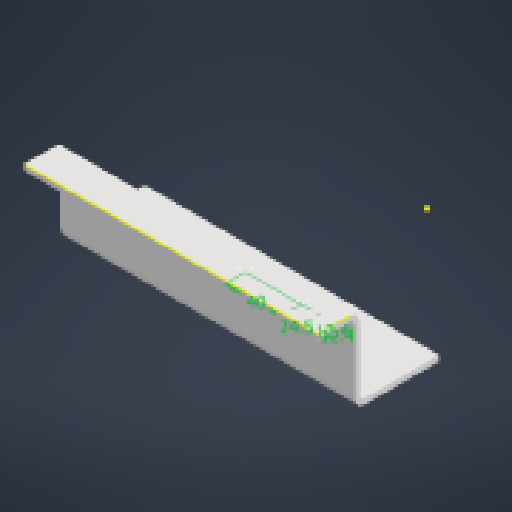
# Autodesk Inventor part: Bottom joint housing R
Saved by Autodesk Inventor 2026.3 (Build 303398000, 398)
## iProperties
Created: 2026-08-05
Part Number: Bottom joint housing R
Material: Generic
Document SubType Name: Sheet Metal
Designer: matot
Density: 1 g/cm^3
Sheet Metal Rule: Default_mm
Appearance: Default
Author: matot
Autodesk Inventor part; units mm, degrees
ref_plane "YZ Plane" through (0, 0, 0) normal (1, 0, 0) x (0, 1, 0)
ref_plane "XZ Plane" through (0, 0, 0) normal (0, 1, 0) x (-1, 0, 0)
ref_plane "XY Plane" through (0, 0, 0) normal (0, 0, 1) x (1, 0, 0)
sketch "Sketch1" plane through (0, 0, 0) normal (0, 1, 0) x (-1, 0, 0)
  line L0 (171.8333, 340.8333) -> (-39.1667, 340.8333)
  line L1 (-39.1667, 340.8333) -> (-39.1667, -59.1667)
  line L2 (-39.1667, -59.1667) -> (171.8333, -59.1667)
  line L3 (171.8333, -59.1667) -> (171.8333, 340.8333)
  point P0 (0, 0)
  dimension "d0" = 400
  dimension "d1" = 211
  measures "d0" distance of L0.end L1.end
  measures "d1" distance of L1.end L2.end
extrude "Plate1" add sketch "Sketch1" along normal blind 4
sketch "Sketch2" plane through (0, 4, 0) normal (0, 1, 0) x (1, 0, 0)
  line L0 (-171.8333, 59.1667) -> (-171.8333, -340.8333) projected
  line L1 (-171.8333, -137.1069) -> (39.1667, -137.1069)
  line L2 (-171.8333, -37.1069) -> (39.1667, -37.1069)
  line L3 (39.1667, -37.1069) -> (39.1667, -37.1069)
  line L4 (39.1667, 59.1667) -> (39.1667, -340.8333) projected
  point P0 (0, 0)
  dimension "d3" = 100
  dimension "d4" = 211
  dimension "d5" = 211
  constraints: 6 end point, 3 perpendicular, 2 point on line, 1 horizontal
  measures "d3" distance between parallel lines of L2 L1
  measures "d4" distance of L2.start L2.end
  measures "d5" distance of L1.start L1.end
fold "Fold1" angle 90 bend radius 4 thickness 4 k factor 0.44 line from (-171.8333, 4, 37.1069) to (39.1667, 4, 37.1069) line at bend centre moving side (0, 0, -1) folds toward (0, 1, 0)
sketch "Sketch3" plane through (0, 0, 0) normal (0, -1, 0) x (1, 0, 0)
  line L0 (39.1667, 41.6308) -> (39.1667, 340.8333) projected
  line L1 (39.1667, 90.6308) -> (-171.8333, 90.6308)
  line L2 (39.1667, 33.6308) -> (-171.8333, 33.6308) projected
  point P0 (0, 0)
  dimension "d12" = 211
  dimension "d13" = 57
  constraints: 2 end point, 1 horizontal, 1 point on line
  measures "d12" distance of L1.start L1.end
  measures "d13" distance between parallel lines of L2 L1
fold "Fold2" angle 90 bend radius 4 thickness 4 k factor 0.44 line from (39.1667, 0, 90.6308) to (-171.8333, 0, 90.6308) line at bend centre moving side (0, 0, -1) folds toward (0, -1, 0)
sketch "Sketch4" plane through (0, 4, 0) normal (0, 1, 0) x (1, 0, 0)
  line L0 (-171.8333, -340.8333) -> (-171.8333, -95.1547) projected
  line L1 (-171.8333, -117.1547) -> (39.1667, -117.1547)
  line L2 (-171.8333, -87.1547) -> (39.1667, -87.1547) projected
  line L3 (39.1667, -95.1547) -> (39.1667, -340.8333) projected
  line L4 (39.1667, -117.1547) -> (-171.8333, -117.1547)
  line L5 (-171.8333, -117.1547) -> (-171.8333, -340.8333)
  line L6 (-171.8333, -340.8333) -> (39.1667, -340.8333)
  line L7 (39.1667, -340.8333) -> (39.1667, -117.1547)
  point P0 (0, 0)
  point P1 (-66.3333, -87.1547)
  dimension "d20" = 211
  dimension "d21" = 30
  constraints: 10 end point, 2 horizontal, 2 parallel, 2 perpendicular, 1 midpoint, 1 point on line
  measures "d20" distance of L1.start L1.end
  measures "d21" distance from line of point (-66.333, -87.155) L1
extrude "Cut1" cut sketch "Sketch4" against normal through all
sketch "Sketch5" plane through (-171.8333, -56.4761, -8.595) normal (0, -1, 0) x (1, 0, 0)
  line L0 (0, 0) -> (0, 91.7497) projected
  line L1 (0, 38.7497) -> (211, 38.7497)
  line L2 (0, 99.7497) -> (211, 99.7497) projected
  line L3 (211, 91.7497) -> (211, 0) projected
  line L4 (211, 0) -> (0, 0) projected
  line L5 (211, 38.7497) -> (0, 38.7497)
  line L6 (0, 38.7497) -> (0, 0)
  line L7 (0, 0) -> (211, 0)
  line L8 (211, 0) -> (211, 38.7497)
  point P0 (171.8333, 8.595)
  dimension "d24" = 211
  dimension "d25" = 61
  constraints: 10 end point, 2 horizontal, 2 parallel, 2 perpendicular, 1 point on line
  measures "d24" distance of L1.start L1.end
  measures "d25" distance between parallel lines of L2 L1
extrude "Cut2" cut sketch "Sketch5" against normal through all
sketch "Sketch6" plane through (-171.8333, -56.4761, 83.1547) normal (0, -1, 0) x (1, 0, 0)
  line L0 (0, -53) -> (211, -53) projected
  line L1 (0, -53) -> (0, 0) projected
  point P0 (171.8333, -83.1547)
  point P1 (66, -26.25)
  point P2 (137.2, -26.25)
  dimension "d28" = 26.75
  dimension "d29" = 26.75
  dimension "d30" = 71.2
  dimension "d31" = 66
  measures "d28" distance from line of L0 point (66, -26.25)
  measures "d29" distance from line of L0 point (137.2, -26.25)
  measures "d30" distance of point (137.2, -26.25) point (66, -26.25)
  measures "d31" distance from line of L1 point (66, -26.25)
hole "Hole1" at (-105.8333, -56.4761, 56.9047) at (-34.6333, -56.4761, 56.9047) direction (0, 1, 0) diameter 3.242 end through all thread size "M4x0.7" class "6H" standard "ISO Metric profile"
sketch "Sketch7" plane through (-171.8333, -56.4761, 83.1547) normal (0, -1, 0) x (1, 0, 0)
  line L0 (0, -53) -> (211, -53) projected
  circle A0 centre (66, -26.25) radius 1.621 projected
  point P0 (171.8333, -83.1547)
  point P1 (84.1, -35.5)
  point P2 (119.1, -35.5)
  dimension "d39" = 17.5
  dimension "d40" = 17.5
  dimension "d41" = 35
  dimension "d42" = 18.1
  measures "d39" distance from line of point (84.1, -35.5) L0
  measures "d40" distance from line of L0 point (119.1, -35.5)
  measures "d41" distance of point (119.1, -35.5) point (84.1, -35.5)
  measures "d42" horizontal distance of point (84.1, -35.5) A0.centre
hole "Hole2" at (-87.7333, -56.4761, 47.6547) at (-52.7333, -56.4761, 47.6547) direction (0, 1, 0) diameter 3.242 end through all thread size "M4x0.7" class "6H" standard "ISO Metric profile"
sketch "Sketch8" plane through (0, 4, 0) normal (0, 1, 0) x (1, 0, 0)
  line L0 (39.1667, -95.1547) -> (39.1667, -117.1547) projected
  line L1 (-171.8333, -117.1547) -> (39.1667, -117.1547) projected
  point P0 (0, 0)
  point P1 (14.6667, -104.9997)
  point P2 (-25.3333, -104.9997)
  dimension "d50" = 40
  dimension "d51" = 24.5
  dimension "d52" = 12.155
  dimension "d53" = 12.155
  measures "d50" distance of point (-25.333, -105) point (14.667, -105)
  measures "d51" distance from line of L0 point (14.667, -105)
  measures "d52" distance from line of L1 point (14.667, -105)
  measures "d53" distance from line of L1 point (-25.333, -105)
hole "Hole3" at (14.6667, 4, 104.9997) at (-25.3333, 4, 104.9997) direction (0, -1, 0) diameter 8.376 end through all thread size "M10x1.5" class "6H" standard "ISO Metric profile"
sketch "Sketch9" plane through (0, 4, 0) normal (0, 1, 0) x (1, 0, 0)
  line L0 (-171.8333, -117.1547) -> (-171.8333, -95.1547) projected
  line L1 (-171.8333, -117.1547) -> (39.1667, -117.1547) projected
  point P0 (0, 0)
  point P1 (-111.8333, -104.9997)
  point P2 (-151.8333, -104.9997)
  point P3 (-171.8333, -106.1547)
  dimension "d61" = 40
  dimension "d62" = 20
  dimension "d63" = 12.155
  dimension "d64" = 12.155
  constraints: 1 midpoint
  measures "d61" distance of point (-151.833, -105) point (-111.833, -105)
  measures "d62" horizontal distance of point (-171.833, -106.155) point (-151.833, -105)
  measures "d63" distance from line of L1 point (-151.833, -105)
  measures "d64" distance from line of L1 point (-111.833, -105)
hole "Hole4" at (-111.8333, 4, 104.9997) at (-151.8333, 4, 104.9997) direction (0, -1, 0) diameter 8.376 end through all thread size "M10x1.5" class "6H" standard "ISO Metric profile"
equation "\"d2\" = Thickness"
equation "\"d6\" = BendReliefWidth"
equation "\"d7\" = BendReliefDepth"
equation "\"d8\" = MinimumRemnant"
equation "\"d9\" = TransitionRadius"
equation "\"d11\" = BendRadius"
equation "\"d14\" = BendReliefWidth"
equation "\"d15\" = BendReliefDepth"
equation "\"d16\" = MinimumRemnant"
equation "\"d17\" = TransitionRadius"
equation "\"d19\" = BendRadius"
equation "\"d22\" = Thickness"
equation "\"d26\" = Thickness"
equation "\"d37\" = Thickness"
equation "\"d59\" = Thickness"
equation "\"BendRadius\" = Thickness"
equation "\"BendReliefWidth\" = Thickness"
equation "\"BendReliefDepth\" = 0.5 * Thickness"
equation "\"CornerReliefSize\" = 4 * Thickness"
equation "\"MinimumRemnant\" = 2 * Thickness"
equation "\"TransitionRadius\" = BendRadius"
equation "\"JacobiRadiusSize\" = BendRadius"
equation "\"GapSize\" = Thickness"
equation "\"Thickness\" = 4"
body "Solid1"
